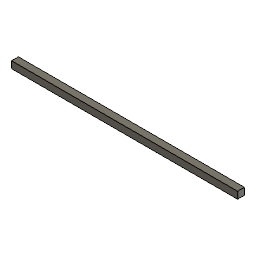
Toothpick (Autodesk Fusion 360 design; units mm, degrees)
part number: 2026-05-31-18-42-09-372
Autodesk Fusion 360 part; units mm, degrees
sketch "Sketch1" plane through (0, 0, 0) normal (0, 1, 0) x (1, 0, 0)
  line L0 (0, 0) -> (65, 0)
  line L1 (0, 0) -> (0, 2)
  line L2 (0, 2) -> (65, 2)
  line L3 (65, 2) -> (65, 0)
  dimension "d1" = 65
  dimension "d2" = 2
  constraint coincident L0.start L1.start
  constraint horizontal L0
  constraint perpendicular L0 L1
  constraint perpendicular L1 L2
  measures "d1" distance of L0.start L0.end
  measures "d2" distance of L0.start L1.end
extrude "Extrude1" add sketch "Sketch1" along normal blind 2
